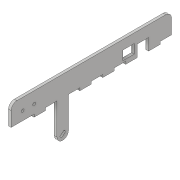
# Autodesk Inventor part: wall
Saved by Autodesk Inventor 2017 (Build 210142000, 142)
## iProperties
Created: 2019-06-11
Part Number: wall
Material: Generic
Document SubType Name: Modeling
Designer: markg
Density: 1 g/cm^3
Appearance: Default
Author: markg
Autodesk Inventor part; units mm, degrees
ref_plane "YZ Plane" through (0, 0, 0) normal (1, 0, 0) x (0, 1, 0)
ref_plane "XZ Plane" through (0, 0, 0) normal (0, 1, 0) x (-1, 0, 0)
ref_plane "XY Plane" through (0, 0, 0) normal (0, 0, 1) x (1, 0, 0)
sketch "Sketch1" plane through (0, 0, 0) normal (1, 0, 0) x (0, 1, 0)
  line L0 (0, 80.3974) -> (25.4, 80.3974)
  line L1 (25.4, 80.3974) -> (25.4, -97.4026)
  line L2 (25.4, -97.4026) -> (0, -97.4026)
  line L3 (0, -97.4026) -> (0, 80.3974)
  point P0 (0, 0)
  dimension "d0" = 177.8
  dimension "d1" = 25.4
  dimension "d2" = 0
  constraints: 8 end point, 2 parallel, 1 horizontal, 1 perpendicular
  measures "d0" distance of L0.end L1.end
  measures "d1" distance of L0.start L0.end
  measures "d2" distance from line of L3 point (0, 0)
extrude "Extrusion1" add sketch "Sketch1" along normal blind 2.921
sketch "Sketch2" plane through (2.921, 0, 0) normal (1, 0, 0) x (0, 0, -1)
  line L0 (-80.3974, 0) -> (97.4026, 0) projected
  line L1 (-67.6974, 0) -> (-54.9974, 0)
  line L2 (-54.9974, 0) -> (-54.9974, 2.921)
  line L3 (-54.9974, 2.921) -> (-67.6974, 2.921)
  line L4 (-67.6974, 2.921) -> (-67.6974, 0)
  line L5 (-80.3974, 25.4) -> (-80.3974, 0) projected
  line L6 (-42.2974, 0) -> (-29.5974, 0)
  line L7 (-29.5974, 0) -> (-29.5974, 2.921)
  line L8 (-29.5974, 2.921) -> (-42.2974, 2.921)
  line L9 (-42.2974, 2.921) -> (-42.2974, 0)
  line L10 (-16.8974, 0) -> (-4.1974, 0)
  line L11 (-4.1974, 0) -> (-4.1974, 2.921)
  line L12 (-4.1974, 2.921) -> (-16.8974, 2.921)
  line L13 (-16.8974, 2.921) -> (-16.8974, 0)
  line L14 (8.5026, 0) -> (21.2026, 0)
  line L15 (21.2026, 0) -> (21.2026, 2.921)
  line L16 (21.2026, 2.921) -> (8.5026, 2.921)
  line L17 (8.5026, 2.921) -> (8.5026, 0)
  line L18 (33.9026, 0) -> (46.6026, 0)
  line L19 (46.6026, 0) -> (46.6026, 2.921)
  line L20 (46.6026, 2.921) -> (33.9026, 2.921)
  line L21 (33.9026, 2.921) -> (33.9026, 0)
  line L22 (59.3026, 0) -> (72.0026, 0)
  line L23 (72.0026, 0) -> (72.0026, 2.921)
  line L24 (72.0026, 2.921) -> (59.3026, 2.921)
  line L25 (59.3026, 2.921) -> (59.3026, 0)
  line L26 (84.7026, 0) -> (97.4026, 0)
  line L27 (97.4026, 0) -> (97.4026, 2.921)
  line L28 (97.4026, 2.921) -> (84.7026, 2.921)
  line L29 (84.7026, 2.921) -> (84.7026, 0)
  point P0 (0, 0)
  dimension "d5" = 12.7
  dimension "d6" = 2.921
  dimension "d7" = 12.7
  dimension "d10" = 25.4
  constraints: 56 end point, 2 horizontal, 2 parallel, 1 collinear, 1 perpendicular, 1 point on line, 47 other
  measures "d5" distance of L2.end L3.end
  measures "d6" distance of L3.end L1.start
  measures "d7" distance between parallel lines of L4 L5
  measures "d10" distance of L1.start L6.start
extrude "Extrusion2" cut sketch "Sketch2" against normal blind 2.921
sketch "Sketch3" plane through (2.921, 0, 0) normal (1, 0, 0) x (0, 0, -1)
  line L0 (-67.6974, 2.921) -> (-67.6974, 0) projected
  line L1 (-80.3974, 25.4) -> (-80.3974, 0) projected
  line L2 (-67.6974, 2.921) -> (-80.3974, 2.921)
  line L3 (-80.3974, 2.921) -> (-80.3974, 0)
  line L4 (-80.3974, 0) -> (-67.6974, 0)
  line L5 (-67.6974, 0) -> (-67.6974, 2.921)
  point P0 (0, 0)
  constraints: 8 end point, 2 parallel, 1 horizontal, 1 perpendicular
extrude "Extrusion3" cut sketch "Sketch3" against normal blind 25.4
sketch "Sketch4" plane through (0, 0, 16.8974) normal (0, -1, 0) x (1, 0, 0)
  line L0 (2.921, 12.7) -> (0, 12.7) projected
  line L1 (0, 0) -> (0, 12.7) projected
  line L2 (0, 0) -> (2.921, 0) projected
  line L3 (2.921, 12.7) -> (2.921, 0) projected
  point P0 (0, -16.8974)
extrude "Extrusion4" add sketch "Sketch4" along normal blind 38.1
fillet "Fillet1" radius 6.35 2 edges at (1.4605, -38.1, 29.5974) (1.4605, -38.1, 16.8974)
sketch "Sketch5" plane through (2.921, 0, 0) normal (1, 0, 0) x (0, 0, -1)
  line L0 (-21.754, -28.8443) -> (-26.6184, -32.926)
  line L1 (-26.6184, -32.926) -> (-24.7408, -35.1637)
  line L2 (-24.7408, -35.1637) -> (-19.8764, -31.082)
  line L3 (-19.8764, -31.082) -> (-21.754, -28.8443)
  line L4 (-21.754, -28.8443) -> (-24.7408, -35.1637) construction
  line L5 (-26.6184, -32.926) -> (-19.8764, -31.082) construction
  line L6 (-16.8974, 2.921) -> (-16.8974, -31.75) projected
  line L7 (-16.8974, 2.921) -> (-4.1974, 2.921) projected
  point P0 (0, 0)
  point P1 (-23.2474, -32.004)
  dimension "d22" = 6.35
  dimension "d23" = 2.921
  dimension "d24" = 6.35
  dimension "d25" = 34.925
  dimension "d29" = 40
  constraints: 12 end point, 2 midpoint, 2 parallel, 1 perpendicular
  measures "d22" distance between parallel lines of L1 L3
  measures "d23" distance between parallel lines of L0 L2
  measures "d24" distance from line of point (-23.247, -32.004) L6
  measures "d25" distance from line of point (-23.247, -32.004) L7
  measures "d29" angle of L7 L0
extrude "Extrusion5" cut sketch "Sketch5" against normal blind 38.1
sketch "Sketch6" plane through (0, 0, 0) normal (-1, 0, 0) x (0, 0, 1)
  circle A0 centre (67.6974, 12.7) radius 1.5875
  circle A1 centre (54.9974, 12.7) radius 1.5875
  line L0 (80.3974, 25.4) -> (-97.4026, 25.4) projected
  line L1 (80.3974, 2.921) -> (80.3974, 25.4) projected
  point P0 (0, 0)
  dimension "d30" = 3.175
  dimension "d31" = 3.175
  dimension "d32" = 12.7
  dimension "d33" = 12.7
  dimension "d34" = 12.7
  dimension "d35" = 12.7
  constraints: 2 centre point
  measures "d30" diameter of A0
  measures "d31" diameter of A1
  measures "d32" distance from line of L0 A0.centre
  measures "d33" distance from line of L0 A1.centre
  measures "d34" distance of A0.centre A1.centre
  measures "d35" distance from line of L1 A0.centre
extrude "Extrusion6" cut sketch "Sketch6" against normal blind 38.1
fillet "Fillet2" radius 6.35 2 edges at (1.4605, 25.4, -97.4026) (1.4605, 25.4, 80.3974)
sketch "Sketch7" plane through (2.921, 0, 0) normal (1, 0, 0) x (0, 0, -1)
  line L0 (59.3026, 2.921) -> (72.0026, 2.921)
  line L1 (72.0026, 2.921) -> (72.0026, 13.081)
  line L2 (72.0026, 13.081) -> (59.3026, 13.081)
  line L3 (59.3026, 13.081) -> (59.3026, 2.921)
  point P0 (0, 0)
  dimension "d39" = 12.7
  dimension "d40" = 10.16
  constraints: 8 end point, 2 parallel, 1 horizontal, 1 perpendicular
  measures "d39" distance of L2.end L1.end
  measures "d40" distance of L1.end L0.end
extrude "Extrusion7" cut sketch "Sketch7" against normal blind 25.4
sketch "Sketch9" plane through (2.921, 0, 0) normal (1, 0, 0) x (0, 0, -1)
  line L0 (56.1276, 15.24) -> (43.4276, 15.24)
  line L1 (43.4276, 15.24) -> (43.4276, 5.08)
  line L2 (43.4276, 5.08) -> (56.1276, 5.08)
  line L3 (56.1276, 5.08) -> (56.1276, 15.24)
  line L4 (59.3026, 0) -> (59.3026, 13.081) projected
  line L5 (97.4026, 2.921) -> (97.4026, 19.05) projected
  line L6 (46.6026, 0) -> (59.3026, 0) projected
  point P0 (0, 0)
  dimension "d43" = 3.175
  dimension "d44" = 53.975
  dimension "d45" = 10.16
  dimension "d46" = 5.08
  constraints: 8 end point, 2 parallel, 1 horizontal, 1 perpendicular
  measures "d43" distance between parallel lines of L4 L3
  measures "d44" distance between parallel lines of L5 L1
  measures "d45" distance of L0.end L1.end
  measures "d46" distance between parallel lines of L6 L2
extrude "Extrusion8" cut sketch "Sketch9" against normal blind 25.4
body "Solid1"
